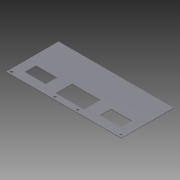
# Autodesk Inventor part: ChassisFrontPlate
Saved by Autodesk Inventor 2012 (Build 160160000, 160)
## iProperties
Created: 2012-04-02
Part Number: ChassisFrontPlate
Material: Steel
Document SubType Name: Modeling
Designer: Jaime
Density: 7.85 g/cm^3
Mass: 86.7832 g
Surface Area: 298.564 cm^2
Volume: 11.0552 cm^3
Author: Jaime
Autodesk Inventor part; units mm, degrees
ref_plane "YZ Plane" through (0, 0, 0) normal (1, 0, 0) x (0, 1, 0)
ref_plane "XZ Plane" through (0, 0, 0) normal (0, 1, 0) x (-1, 0, 0)
ref_plane "XY Plane" through (0, 0, 0) normal (0, 0, 1) x (1, 0, 0)
sketch "Sketch1" plane through (0, 0, 0) normal (0, 0, 1) x (1, 0, 0)
  line L0 (0, 0) -> (195.58, 0)
  line L1 (195.58, 0) -> (195.58, -88.9)
  line L2 (195.58, -88.9) -> (0, -88.9)
  line L3 (0, -88.9) -> (0, 0)
  dimension "d0" = 195.58
  dimension "d1" = 88.9
  constraints: 8 end point, 2 parallel, 1 horizontal, 1 perpendicular
  measures "d0" distance of L0.start L0.end
  measures "d1" distance of L2.end L0.start
extrude "Extrusion1" add sketch "Sketch1" along normal blind 0.762
sketch "Sketch9" plane through (0, 0, 0.762) normal (0, 0, 1) x (1, 0, 0)
  line L0 (195.58, 0) -> (195.58, -88.9) projected
  line L1 (0, -88.9) -> (0, 0) projected
  line L2 (195.58, -88.9) -> (0, -88.9) projected
  line L3 (16.256, -54.61) -> (51.816, -54.61)
  line L4 (51.816, -54.61) -> (51.816, -73.66)
  line L5 (51.816, -73.66) -> (16.256, -73.66)
  line L6 (16.256, -73.66) -> (16.256, -54.61)
  line L7 (143.764, -54.61) -> (179.324, -54.61)
  line L8 (179.324, -54.61) -> (179.324, -73.66)
  line L9 (179.324, -73.66) -> (143.764, -73.66)
  line L10 (143.764, -73.66) -> (143.764, -54.61)
  line L11 (73.66, -50.8) -> (121.92, -50.8)
  line L12 (121.92, -50.8) -> (121.92, -78.74)
  line L13 (121.92, -78.74) -> (73.66, -78.74)
  line L14 (73.66, -78.74) -> (73.66, -50.8)
  dimension "d105" = 16.256
  dimension "d106" = 19.05
  dimension "d107" = 35.56
  dimension "d108" = 16.256
  dimension "d109" = 19.05
  dimension "d110" = 35.56
  dimension "d111" = 15.24
  dimension "d112" = 15.24
  dimension "d113" = 48.26
  dimension "d114" = 27.94
  dimension "d115" = 73.66
  dimension "d116" = 73.66
  dimension "d117" = 10.16
  constraints: 24 end point, 6 parallel, 3 horizontal, 3 perpendicular
  measures "d105" distance between parallel lines of L6 L1
  measures "d106" distance between parallel lines of L3 L5
  measures "d107" distance between parallel lines of L6 L4
  measures "d108" distance between parallel lines of L0 L8
  measures "d109" distance between parallel lines of L7 L9
  measures "d110" distance between parallel lines of L8 L10
  measures "d111" distance between parallel lines of L2 L5
  measures "d112" distance between parallel lines of L2 L9
  measures "d113" distance between parallel lines of L12 L14
  measures "d114" distance between parallel lines of L13 L11
  measures "d115" distance between parallel lines of L1 L14
  measures "d116" distance between parallel lines of L0 L12
  measures "d117" distance between parallel lines of L2 L13
extrude "Extrusion4" cut sketch "Sketch9" against normal blind 25.4
sketch "Sketch10" plane through (0, 0, 0.762) normal (0, 0, 1) x (1, 0, 0)
  circle A0 centre (4.7625, -84.7725) radius 2.2479 projected
  circle A1 centre (78.4225, -84.7725) radius 2.2479 projected
  circle A2 centre (117.1575, -84.7725) radius 2.2479 projected
  circle A3 centre (190.8175, -84.7725) radius 2.2479 projected
  line L0 (195.58, -88.9) -> (0, -88.9) projected
  line L1 (0, -37.5396) -> (9.525, -37.5396) projected
  point P0 (4.7625, -33.02)
  point P1 (4.7625, -7.62)
  point P2 (78.4225, -7.62)
  point P3 (78.4225, -33.02)
  point P4 (117.1575, -33.02)
  point P5 (117.1575, -7.62)
  point P6 (190.8175, -33.02)
  point P7 (190.8175, -7.62)
  dimension "d127" = 81.28
  dimension "d128" = 55.88
  dimension "d129" = 55.88
  dimension "d130" = 81.28
  dimension "d131" = 81.28
  dimension "d132" = 55.88
  dimension "d133" = 55.88
  dimension "d134" = 81.28
  constraints: 4 coincident
  measures "d127" distance from line of point (4.763, -7.62) L0
  measures "d128" distance from line of L0 point (4.763, -33.02)
  measures "d129" distance from line of L0 point (78.423, -33.02)
  measures "d130" distance from line of L0 point (78.423, -7.62)
  measures "d131" distance from line of L0 point (117.157, -7.62)
  measures "d132" distance from line of L0 point (117.157, -33.02)
  measures "d133" distance from line of L0 point (190.817, -33.02)
  measures "d134" distance from line of L0 point (190.817, -7.62)
hole "Hole5" at (190.8175, -84.7725, 0.762) at (117.1575, -84.7725, 0.762) at (78.4225, -84.7725, 0.762) at (4.7625, -84.7725, 0.762) at (4.7625, -7.62, 0.762) at (4.7625, -33.02, 0.762) at (78.4225, -33.02, 0.762) at (78.4225, -7.62, 0.762) at (117.1575, -7.62, 0.762) at (117.1575, -33.02, 0.762) at (190.8175, -33.02, 0.762) at (190.8175, -7.62, 0.762) direction (0, 0, -1) diameter 4.318 end through all clearance for "Flat Head Machine Screw (82)" size "#8" standard "Ansi Unified Screw Threads"
body "Solid1"
